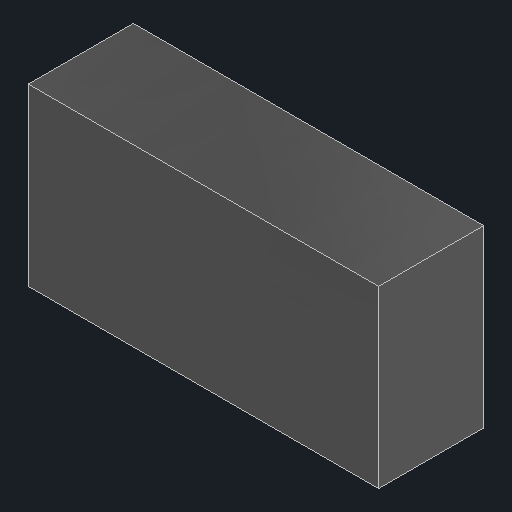
# Autodesk Inventor part: lipo3s650mah
Saved by Autodesk Inventor 2023 (Build 270158000, 158)
## iProperties
Created: 2024-05-25
Part Number: lipo3s650mah
Material: Generic
Document SubType Name: Modeling
Designer: szymo
Density: 1.85185 g/cm^3
Appearance: Dark Gray
Mass: 60 g
Surface Area: 68.4 cm^2
Volume: 32.4 cm^3
TOTAL MASS: 0.0
Author: szymo
Autodesk Inventor part; units mm, degrees
ref_plane "YZ Plane" through (0, 0, 0) normal (1, 0, 0) x (0, 1, 0)
ref_plane "XZ Plane" through (0, 0, 0) normal (0, 1, 0) x (-1, 0, 0)
ref_plane "XY Plane" through (0, 0, 0) normal (0, 0, 1) x (1, 0, 0)
sketch "Sketch1" plane through (0, 0, 0) normal (0, 1, 0) x (-1, 0, 0)
  line L0 (0, 0) -> (-60, 0)
  line L1 (-60, 0) -> (-60, -18)
  line L2 (-60, -18) -> (0, -18)
  line L3 (0, -18) -> (0, 0)
  dimension "d0" = 60
  dimension "d1" = 18
  constraints: 8 end point, 2 parallel, 1 horizontal, 1 perpendicular
  measures "d0" distance of L2.end L1.end
  measures "d1" distance of L1.end L0.end
extrude "Extrusion1" add sketch "Sketch1" along normal blind 30
body "Solid1"
